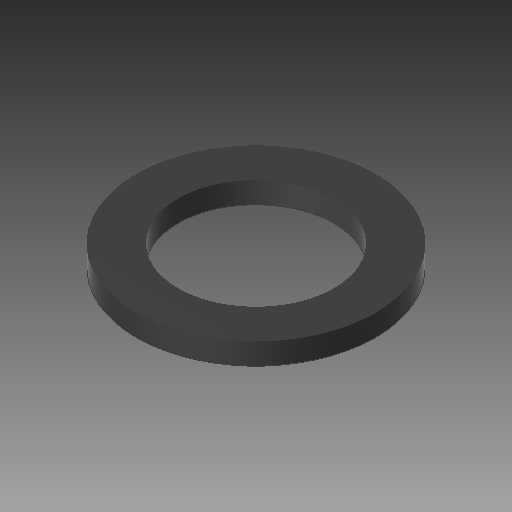
# Autodesk Inventor part: CC-0815-08B
Saved by Autodesk Inventor 2018 (Build 220112000, 112)
## iProperties
Created: 2016-08-26
Part Number: CC-0815-08B
Material: アセタール樹脂、黒
Document SubType Name: Modeling
Designer: hiro
Density: 1.425 g/cm^3
Appearance: 滑らか - 黒
Mass: 0.0774033 g
Surface Area: 1.65813 cm^2
Volume: 0.0543181 cm^3
Author: hiro
Autodesk Inventor part; units mm, degrees
ref_plane "YZ Plane" through (0, 0, 0) normal (1, 0, 0) x (0, 1, 0)
ref_plane "XZ Plane" through (0, 0, 0) normal (0, 1, 0) x (-1, 0, 0)
ref_plane "XY Plane" through (0, 0, 0) normal (0, 0, 1) x (1, 0, 0)
sketch "スケッチ1" plane through (0, 0, 0) normal (0, 0, 1) x (1, 0, 0)
  line L0 (3.6, 0.5) -> (5.5, 0.5)
  line L1 (5.5, 0.5) -> (5.5, -0.5)
  line L2 (5.5, -0.5) -> (3.6, -0.5)
  line L3 (3.6, -0.5) -> (3.6, 0.5)
  line L4 (0, 1.7462) -> (0, -1.7462) construction
  point P0 (0, 0)
  point P1 (0, 0)
  point P2 (3.6, 0)
  dimension "d0" = 1
  dimension "d1" = 7.2
  dimension "d2" = 11
  constraints: 10 end point, 2 midpoint, 2 parallel, 1 coincident, 1 horizontal, 1 horizontal alignment, 1 perpendicular, 1 vertical
  measures "d0" distance of L0.end L1.end
  measures "d1" diameter of L3 L4
  measures "d2" diameter of L1 L4
revolve "回転1" add sketch "スケッチ1" angle 360 about axis through (0, 1.7462, 0) along (0, -1, 0)
